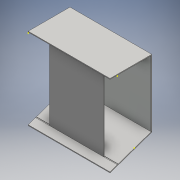
# Autodesk Inventor part: zderzaki
Saved by Autodesk Inventor 2016 (Build 200138000, 138)
## iProperties
Created: 2015-11-10
Part Number: zderzaki
Material: Ogólny
Document SubType Name: Modeling
Designer: Mrianura
Density: 1 g/cm^3
Appearance: Domyślna
Author: Mrianura
Autodesk Inventor part; units mm, degrees
ref_plane "YZ Plane" through (0, 0, 0) normal (1, 0, 0) x (0, 1, 0)
ref_plane "XZ Plane" through (0, 0, 0) normal (0, 1, 0) x (-1, 0, 0)
ref_plane "XY Plane" through (0, 0, 0) normal (0, 0, 1) x (1, 0, 0)
sketch "Szkic1" plane through (0, 0, 0) normal (1, 0, 0) x (0, 1, 0)
  line L0 (0, 0) -> (0, -88)
  line L1 (51.058, -70.4193) -> (51.058, -71.4193)
  line L2 (0, -88) -> (0, -97)
  line L3 (0, -97) -> (0, -98)
  line L4 (0, -98) -> (51.058, -80.4193)
  line L5 (51.058, -80.4193) -> (51.058, -79.4193)
  line L6 (51.058, -79.4193) -> (0, -97)
  line L7 (0, 0) -> (0, 1)
  line L8 (0, 1) -> (51.058, 1)
  line L9 (51.058, 1) -> (51.058, 2)
  line L10 (51.058, 2) -> (0, 2)
  line L11 (0, 2) -> (0, 1)
  dimension "d0" = 88
  dimension "d1" = 54
  dimension "d5" = 9
  dimension "d6" = 1
  dimension "d7" = 54
  dimension "d8" = 71
  dimension "d9" = 1
  dimension "d10" = 1
  dimension "d11" = 1
  constraints: 24 end point, 5 point on line, 3 perpendicular, 3 vertical, 1 parallel
  measures "d0" distance of L0.start L0.end
  measures "d1" distance of L0.end L1.start
  measures "d5" distance of L0.end L2.end
  measures "d6" distance of L2.end L3.end
  measures "d7" distance of L3.end L4.end
  measures "d8" angle of L4 L3
  measures "d9" distance of L4.end L5.end
  measures "d10" distance of L0.start L7.end
  measures "d11" distance of L8.end L9.end
extrude "Wyciągnięcie proste1" add sketch "Szkic1" against normal blind 100
sketch "Szkic2" plane through (-100, 0, 0) normal (-1, 0, 0) x (0, 0, 1)
  line L0 (0, 10) -> (1, 10)
  line L1 (1, 51.058) -> (1, 0) projected
  line L2 (0, 10) -> (-93.5567, 10)
  line L3 (-79.4193, 51.058) -> (-97, 0) projected
  line L4 (0, 9) -> (1, 9)
  line L5 (0, 9) -> (-93.9011, 9)
  line L6 (-93.5567, 10) -> (-93.9011, 9)
  line L7 (1, 10) -> (1, 9)
  point P0 (0, 0)
  dimension "d14" = 10
  dimension "d15" = 1
  constraints: 12 end point, 5 point on line, 2 collinear, 1 horizontal, 1 perpendicular
  measures "d14" distance of point (0, 0) L0.start
  measures "d15" distance of L0.start L4.start
extrude "Wyciągnięcie proste2" add sketch "Szkic2" against normal blind 100
sketch "Szkic3" plane through (-100, 51.058, -79.4193) normal (0, -0.3255682, 0.9455186) x (1, 0, 0)
  point P0 (100, -22.4199)
sketch "Szkic4" plane through (-100, 51.058, -80.4193) normal (0, 1, 0) x (1, 0, 0)
  line L0 (100, -81.4193) -> (100, 13.4817) projected
  line L1 (100, 0) -> (100, -1) projected
  line L2 (100, -81.4193) -> (100, -1)
  line L3 (0, -1) -> (0, 0) projected
  line L4 (100, -1) -> (0, -1)
  line L5 (0, 13.4817) -> (0, -81.4193) projected
  line L6 (0, -1) -> (0, -81.4193)
  line L7 (100, -81.4193) -> (0, -81.4193) projected
  line L8 (0, -81.4193) -> (100, -81.4193)
  point P0 (100, -80.4193)
  constraints: 8 end point, 3 collinear, 1 perpendicular
extrude "Wyciągnięcie proste3" add sketch "Szkic4" against normal blind 1
sketch "Szkic5" plane through (-100, 9, -93.9011) normal (0, -1, 0) x (1, 0, 0)
  point P0 (100, 93.9011)
sketch "Szkic6" plane through (-100, 51.058, -79.4193) normal (-1, 0, 0) x (0, 0, -1)
  point P0 (-79.4193, 51.058)
sketch "Szkic7" plane through (-100, 9, -93.9011) normal (0, -1, 0) x (1, 0, 0)
  line L0 (100, 14.4817) -> (100, 94.9011) projected
  line L1 (100, 94.9011) -> (90, 94.9011)
  line L2 (0, 94.9011) -> (100, 94.9011) projected
  line L3 (90, 94.9011) -> (90, 0)
  line L4 (100, 0) -> (0, 0) projected
  line L5 (90, 0) -> (100, 0)
  line L6 (100, 0) -> (100, 94.9011)
  line L7 (90, 94.9011) -> (100, 94.9011)
  line L8 (0, 94.9011) -> (10, 94.9011)
  line L9 (10, 94.9011) -> (10, 0)
  line L10 (0, 0) -> (0, 94.9011) projected
  line L11 (10, 0) -> (0, 0)
  line L12 (0, 94.9011) -> (0, 14.4817) projected
  line L13 (0, 0) -> (0, 94.9011)
  line L14 (0, 94.9011) -> (10, 94.9011)
  point P0 (100, 93.9011)
  dimension "d20" = 10
  dimension "d21" = 10
  constraints: 20 end point, 4 collinear, 4 point on line, 3 perpendicular, 1 horizontal
  measures "d20" distance of L0.end L1.end
  measures "d21" distance of L2.start L8.end
extrude "Wyciągnięcie proste4" cut sketch "Szkic7" against normal blind 1 contours L6 L4 L3 L1 L0 | L9 L4 L10 L2
sketch "Szkic8" plane through (-90, 9, 1) normal (0, -1, 0) x (1, 0, 0)
  line L0 (80, -94.9011) -> (80, 0) projected
  line L1 (80, 0) -> (73, 0)
  line L2 (80, 0) -> (0, 0) projected
  line L3 (73, 0) -> (73, -94.9011)
  line L4 (80, -94.9011) -> (0, -94.9011) projected
  line L5 (80, -94.9011) -> (80, 0)
  line L6 (90, 1) -> (-10, 1) projected
  line L7 (80, 0) -> (73, 0)
  line L8 (0, 0) -> (7, 0)
  line L9 (7, 0) -> (7, -94.9011)
  line L10 (0, -94.9011) -> (7, -94.9011)
  line L11 (0, 0) -> (0, -94.9011) projected
  line L12 (0, -94.9011) -> (0, 0)
  line L13 (0, -94.5567) -> (0, 0) projected
  point P0 (90, -1)
  dimension "d24" = 7
  dimension "d25" = 7
  constraints: 16 end point, 4 point on line, 3 collinear, 3 perpendicular
  measures "d24" distance of L0.end L1.end
  measures "d25" distance of L2.end L8.end
extrude "Wyciągnięcie proste5" cut sketch "Szkic8" against normal blind 1 contours L4 L3 L1 L0 | L4 L11 L2 L9
